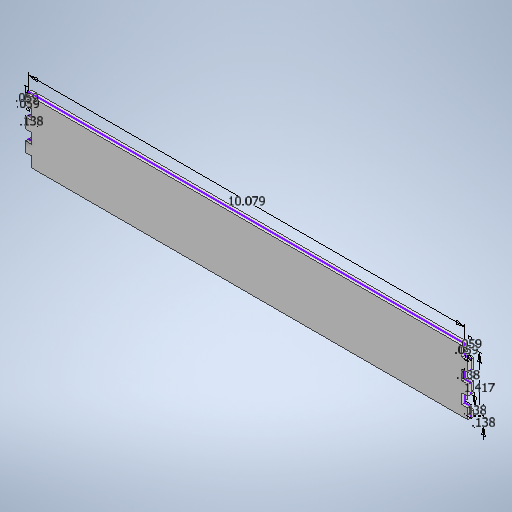
# Autodesk Inventor part: Side Wall 3
Saved by Autodesk Inventor 2025.3 (Build 293356000, 356)
## iProperties
Created: 2025-04-23
Part Number: Side Wall 3
Material: Generic
Document SubType Name: Modeling
Designer: powel
Density: 1 g/cm^3
Appearance: Default
Author: powel
Autodesk Inventor part; units mm, degrees
ref_plane "YZ Plane" through (0, 0, 0) normal (1, 0, 0) x (0, 1, 0)
ref_plane "XZ Plane" through (0, 0, 0) normal (0, 1, 0) x (-1, 0, 0)
ref_plane "XY Plane" through (0, 0, 0) normal (0, 0, 1) x (1, 0, 0)
sketch "Sketch1" plane through (0, 0, 0) normal (0, 0, 1) x (1, 0, 0)
  line L0 (3.5, 0) -> (256, 0)
  line L1 (256, 36) -> (0, 36)
  line L2 (256, 36) -> (256, 30)
  line L3 (256, 24) -> (256, 18)
  line L4 (256, 12) -> (256, 6)
  line L5 (256, 30) -> (259.5, 30)
  line L6 (259.5, 30) -> (259.5, 24)
  line L7 (259.5, 24) -> (256, 24)
  line L8 (256, 18) -> (259.5, 18)
  line L9 (259.5, 18) -> (259.5, 12)
  line L10 (259.5, 12) -> (256, 12)
  line L11 (256, 6) -> (259.5, 6)
  line L12 (259.5, 6) -> (259.5, 0)
  line L13 (259.5, 0) -> (256, 0)
  line L14 (0, 36) -> (0, 30)
  line L15 (0, 24) -> (0, 18)
  line L16 (0, 12) -> (0, 6)
  line L17 (0, 30) -> (3.5, 30)
  line L18 (3.5, 30) -> (3.5, 24)
  line L19 (3.5, 24) -> (0, 24)
  line L20 (0, 18) -> (3.5, 18)
  line L21 (3.5, 18) -> (3.5, 12)
  line L22 (3.5, 12) -> (0, 12)
  line L23 (0, 6) -> (3.5, 6)
  line L24 (3.5, 6) -> (3.5, 0)
  line L25 (0, 36) -> (256, 36)
  line L26 (256, 36) -> (256, 34.5)
  line L27 (256, 34.5) -> (0, 34.5)
  line L28 (0, 34.5) -> (0, 36)
  line L29 (256, 34.5) -> (0, 34.5)
  line L30 (0, 34.5) -> (0, 33)
  line L31 (0, 33) -> (256, 33)
  line L32 (256, 33) -> (256, 34.5)
  line L33 (0, 33) -> (256, 33)
  line L34 (256, 33) -> (256, 31.5)
  line L35 (256, 31.5) -> (0, 31.5)
  line L36 (0, 31.5) -> (0, 33)
  line L37 (256, 31.5) -> (0, 31.5)
  line L38 (0, 31.5) -> (0, 30)
  line L39 (0, 30) -> (256, 30)
  line L40 (256, 30) -> (256, 31.5)
  line L41 (259.5, 0) -> (3.5, 0)
  line L42 (3.5, 0) -> (3.5, 3.5)
  line L43 (3.5, 3.5) -> (259.5, 3.5)
  line L44 (259.5, 3.5) -> (259.5, 0)
  line L45 (3.5, 3.5) -> (259.5, 3.5)
  line L46 (259.5, 3.5) -> (259.5, 6)
  line L47 (256, 7) -> (0, 7)
  line L48 (0, 7) -> (0, 6)
  dimension "d52" = 256
  dimension "d53" = 36
  dimension "d60" = 3.5
  dimension "d67" = 3.5
  dimension "d68" = 1.5
  dimension "d69" = 1.5
  dimension "d70" = 1.5
  dimension "d71" = 1.5
  dimension "d74" = 3.5
  dimension "d75" = 3.5
  constraints: 98 end point, 18 parallel, 13 horizontal, 12 perpendicular, 8 point on line, 1 midpoint
  measures "d52" distance of L1.end L1.start
  measures "d53" distance of L1.start L0.end
  measures "d60" distance of L6.end L7.end
  measures "d67" distance of L18.end L19.end
  measures "d68" distance of L25.end L26.end
  measures "d69" distance of L30.end L29.end
  measures "d70" distance of L33.end L34.end
  measures "d71" distance of L14.end L37.end
  measures "d74" distance between parallel lines of L47 L43
  measures "d75" distance between parallel lines of L41 L45
extrude "Extrusion1" add sketch "Sketch1" along normal blind 1.75
extrude "Extrusion2" add sketch "Sketch1" against normal blind 1.75 contours L24 L43 L12 L13 L0 | L16 L22 L21 L20 L15 L19 L18 L39 L5 L6 L7 L3 L8 L9 L10 L4 L47 | L14 L31 L2 L35 | L14 L1 L2 L27
body "Solid1"
